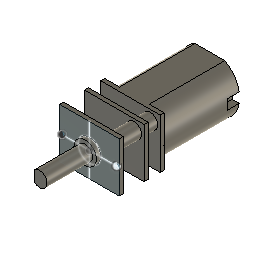
N20 motor (Autodesk Fusion 360 design; units mm, degrees)
Autodesk Fusion 360 part; units mm, degrees
note: some values were not read from the file. Set by a fixed rule: which sketch regions a step uses.
sketch "Sketch1" plane through (0, 0, 0) normal (0, 1, 0) x (1, 0, 0)
  line L0 (0, 0) -> (12, 0)
  line L1 (0, 0) -> (0, -10)
  line L2 (12, 0) -> (12, -10)
  line L3 (12, -10) -> (0, -10)
  line L4 (12, -10) -> (9, -10)
  arc A0 (9, -10) -> (9, 0) centre (6.3333, -5) ccw
  line L5 (0, -10) -> (3, -10)
  arc A1 (3, 0) -> (3, -10) centre (5.6667, -5) ccw
  dimension "d3" = 12
  dimension "d4" = 10
  dimension "d5" = 3
  dimension "d6" = 3
  constraint coincident L0.start L1.start
  constraint horizontal L0
  constraint perpendicular L0 L1
  constraint perpendicular L0 L2
  constraint perpendicular L1 L3
  constraint perpendicular L2 L4
  constraint tangent L2 A0
  constraint coincident L0 A0.end
  constraint perpendicular L1 L5
  constraint tangent L1 A1
  constraint coincident L0 A1.start
  measures "d3" distance of L0.start L0.end
  measures "d4" distance of L0.start L1.end
  measures "d5" distance of L2.end L4.end
  measures "d6" distance of L1.end L5.end
extrude "Extrude1" add sketch "Sketch1" along normal blind 15.2 contours L0 L3 A0 A1 makes body 1
sketch "Sketch2" plane through (0, 0, 0) normal (0, -1, 0) x (1, 0, 0)
  arc A0 (9, 0) -> (9, 10) centre (6.3333, 5) ccw
  line L0 (9, 10) -> (3, 10)
  arc A1 (3, 10) -> (3, 0) centre (5.6667, 5) ccw
  line L1 (3, 0) -> (9, 0)
  line L2 (0, 10) -> (12, 10)
  line L3 (12, 10) -> (12, 0)
  line L4 (12, 0) -> (0, 0)
  line L5 (0, 0) -> (0, 10)
  constraint parallel L0 L2
  constraint perpendicular L2 L3
  constraint coincident L4.end L5.start
  constraint perpendicular L3 L4
  constraint perpendicular L2 L5
extrude "Extrude2" add sketch "Sketch2" along normal blind 0.8 bodies 1
sketch "Sketch3" plane through (0, -0.8, 0) normal (0, -1, 0) x (1, 0, 0)
  line L0 (0, 0) -> (12, 0)
  line L1 (12, 0) -> (12, 10)
  line L2 (12, 10) -> (0, 10)
  line L3 (0, 10) -> (0, 0)
  circle A0 centre (2, 2) radius 1.5
  circle A1 centre (10, 8) radius 1.5
  dimension "d11" = 3
  dimension "d12" = 3
  measures "d11" diameter of A0
  measures "d12" diameter of A1
extrude "Extrude3" add sketch "Sketch3" along normal blind 2.45 contours A0 | A1 bodies 1
sketch "Sketch4" plane through (0, -3.25, 0) normal (0, -1, 0) x (1, 0, 0)
  circle A0 centre (2, 2) radius 1.5
  line L0 (0, 10) -> (12, 10)
  line L1 (12, 10) -> (12, 0)
  line L2 (12, 0) -> (0, 0)
  line L3 (0, 0) -> (0, 10)
  constraint horizontal L0
  constraint vertical L1
  constraint horizontal L2
  constraint vertical L3
extrude "Extrude4" add sketch "Sketch4" along normal blind 0.8 separate body makes body 2
extrude "Extrude5" add 1 faces at (1.5, -3.25, 2.6802) along direction (0, -1, 0) blind 0.8 on bodies 1 bodies 1 2
sketch "Sketch5" plane through (0, -4.05, 0) normal (0, -1, 0) x (1, 0, 0)
  line L0 (0, 0) -> (12, 0)
  line L1 (12, 0) -> (12, 10)
  line L2 (12, 10) -> (0, 10)
  line L3 (0, 10) -> (0, 0)
  circle A0 centre (2, 2) radius 1.5
  circle A1 centre (10, 8) radius 1.5
  dimension "d19" = 3
  dimension "d20" = 3
  measures "d19" diameter of A0
  measures "d20" diameter of A1
extrude "Extrude6" add sketch "Sketch5" along normal blind 4.2 contours A0 | A1 bodies 1
sketch "Sketch6" plane through (0, -8.25, 0) normal (0, -1, 0) x (1, 0, 0)
  circle A0 centre (10, 8) radius 1.5
  line L0 (0, 10) -> (12, 10)
  line L1 (12, 10) -> (12, 0)
  line L2 (12, 0) -> (0, 0)
  line L3 (0, 0) -> (0, 10)
  constraint horizontal L0
  constraint vertical L1
  constraint horizontal L2
  constraint vertical L3
extrude "Extrude7" add sketch "Sketch6" along normal blind 0.8 contours A0 | L0 L1 L2 L3 bodies 1
sketch "Sketch7" plane through (0, -9.05, 0) normal (0, -1, 0) x (1, 0, 0)
  line L0 (0, 0) -> (12, 0)
  line L1 (12, 0) -> (12, 10)
  line L2 (12, 10) -> (0, 10)
  line L3 (0, 10) -> (0, 0)
  line L4 (0, 5) -> (12, 5)
  line L5 (6, 10) -> (6, 0)
  circle A0 centre (6, 5) radius 2.25
  circle A1 centre (0.5, 5) radius 0.35
  circle A2 centre (11.5, 5) radius 0.35
  dimension "d25" = 4.5
  dimension "d26" = 0.7
  constraint midpoint L3 L4.start
  constraint midpoint L1 L4.end
  constraint midpoint L2 L5.start
  constraint midpoint L0 L5.end
  constraint midpoint L4 A0.centre
  constraint coincident L4 A1.centre
  constraint symmetric L5 A1 A2
  measures "d25" diameter of A0
  measures "d26" diameter of A1
extrude "Extrude8" cut sketch "Sketch7" against normal blind 2 contours L4 A1 | L4 A1 | L4 A2 | L4 A2 bodies 1
extrude "Extrude9" add sketch "Sketch7" along normal blind 0.87 contours L4 L5 A0 | L4 L5 A0 | L4 L5 A0 | L4 L5 A0 bodies 1
sketch "Sketch8" plane through (0, -9.92, 0) normal (0, -1, 0) x (1, 0, 0)
  circle A0 centre (6, 5) radius 2.25
  line L0 (7.5, 5) -> (5, 5)
  line L1 (5, 5) -> (5, 6.118)
  line L2 (5, 5) -> (5, 3.882)
  arc A1 (5, 3.882) -> (5, 6.118) centre (6, 5) ccw
  dimension "d31" = 3
  dimension "d32" = 2.5
  constraint concentric A0 A1
  constraint coincident L0.start A1
  constraint horizontal L0
  constraint perpendicular L0 L1
  constraint perpendicular L0 L2
  measures "d31" diameter of A1
  measures "d32" distance of L0.start L0.end
extrude "Extrude10" add sketch "Sketch8" along normal blind 9.17 contours L0 L2 A1 | L0 L1 A1 bodies 1
sketch "Sketch9" plane through (0, 15.2, 0) normal (0, 1, 0) x (-1, 0, 0)
  arc A0 (-9, 10) -> (-9, 0) centre (-6.3333, 5) ccw
  line L0 (-9, 0) -> (-3, 0)
  arc A1 (-3, 0) -> (-3, 10) centre (-5.6667, 5) ccw
  line L1 (-3, 10) -> (-9, 10)
  circle A2 centre (-6, 5) radius 2.5
  line L2 (0, 5) -> (-1.5, 5)
  line L3 (-1.5, 5) -> (-1.5, 4)
  line L4 (0, 5) -> (0, 6)
  line L5 (0, 6) -> (-1.5, 6)
  line L6 (-1.5, 6) -> (-1.5, 4)
  line L7 (-1.5, 4) -> (0, 4)
  line L8 (0, 4) -> (0, 6)
  line L9 (-6, 10) -> (-6, 0)
  line L10 (-10.5, 6) -> (-10.5, 4)
  line L11 (-12, 4) -> (-12, 6)
  line L12 (-10.5, 4) -> (-12, 4)
  line L13 (-12, 6) -> (-10.5, 6)
  dimension "d35" = 5
  dimension "d36" = 1.5
  dimension "d37" = 1
  dimension "d38" = 1
  constraint midpoint A1 L2.start
  constraint horizontal L2
  constraint perpendicular L2 L3
  constraint perpendicular L2 L4
  constraint horizontal L5
  constraint vertical L6
  constraint horizontal L7
  constraint vertical L8
  constraint symmetric L3.end L9 L10.end
  constraint symmetric L4.end L9 L11.end
  constraint symmetric L5.end L9 L10.start
  constraint symmetric L7.end L9 L11.start
  measures "d35" diameter of A2
  measures "d36" distance of L2.start L2.end
  measures "d37" distance of L2.end L3.end
  measures "d38" distance of L2.start L4.end
extrude "Extrude11" add sketch "Sketch9" along normal blind 0.9 contours A2 L9 | A2 L9 bodies 1
extrude "Extrude12" cut sketch "Sketch9" against normal blind 2.37 contours A0 L10 L12 L13 | A1 L2 L5 L6 | A1 L2 L3 L6 L7 bodies 1
sketch "Sketch10" plane through (0, 15.2, 0) normal (0, 1, 0) x (-1, 0, 0)
  line L0 (-0.0889, 4) -> (-1.5, 4)
  line L1 (-1.5, 4) -> (-1.5, 6)
  line L2 (-1.5, 6) -> (-0.0889, 6)
  arc A0 (-0.0889, 6) -> (-3, 10) centre (-5.6667, 5) ccw
  line L3 (-3, 10) -> (-9, 10)
  arc A1 (-9, 10) -> (-11.9111, 6) centre (-6.3333, 5) ccw
  line L4 (-11.9111, 6) -> (-10.5, 6)
  line L5 (-10.5, 6) -> (-10.5, 4)
  line L6 (-10.5, 4) -> (-11.9111, 4)
  arc A2 (-11.9111, 4) -> (-9, 0) centre (-6.3333, 5) ccw
  line L7 (-9, 0) -> (-3, 0)
  arc A3 (-3, 0) -> (-0.0889, 4) centre (-5.6667, 5) ccw
  circle A4 centre (-6, 5) radius 2.5
  line L8 (-3.5, 5) -> (-2.39, 5)
  line L9 (-2.39, 5) -> (-2.39, 4.25)
  line L10 (-2.39, 4.25) -> (-2.09, 4.25)
  line L11 (-2.09, 4.25) -> (-2.09, 5)
  line L12 (0, 5) -> (-12, 5)
  line L13 (-3.5, 5) -> (-2.39, 5)
  line L14 (-2.39, 5.75) -> (-2.09, 5.75)
  line L15 (-2.09, 5.75) -> (-2.09, 5)
  line L16 (-2.39, 5) -> (-2.39, 5.75)
  line L17 (-6, 10) -> (-6, 0)
  line L18 (-9.61, 5) -> (-9.61, 4.25)
  line L19 (-9.91, 4.25) -> (-9.91, 5)
  line L20 (-9.61, 4.25) -> (-9.91, 4.25)
  line L21 (-12, 5) -> (0, 5)
  line L22 (-9.61, 5.75) -> (-9.91, 5.75)
  line L23 (-9.61, 5) -> (-9.61, 5.75)
  line L24 (-9.91, 5.75) -> (-9.91, 5)
  dimension "d43" = 1.11
  dimension "d44" = 0.75
  dimension "d45" = 0.3
  constraint coincident A4 L8.start
  constraint perpendicular L1 L8
  constraint perpendicular L8 L9
  constraint perpendicular L9 L10
  constraint perpendicular L10 L11
  constraint symmetric L8.start L12 L13.start
  constraint symmetric L8.end L12 L9.start
  constraint symmetric L9.end L12 L14.start
  constraint symmetric L10.end L12 L14.end
  constraint symmetric L11.end L12 L15.end
  constraint symmetric L8.end L17 L18.start
  constraint symmetric L9.end L17 L18.end
  constraint symmetric L10.end L17 L19.start
  constraint symmetric L11.end L17 L19.end
  constraint symmetric L12.start L17 L12.end
  constraint symmetric L12.end L17 L12.start
  constraint symmetric L14.start L17 L22.start
  constraint symmetric L14.end L17 L22.end
  measures "d43" distance of L8.start L8.end
  measures "d44" distance of L8.end L9.end
  measures "d45" distance of L9.end L10.end
extrude "Extrude13" add sketch "Sketch10" along normal blind 1.31 contours L9 L10 L11 L12 L21 | L12 L14 L15 L16 L21 | L12 L18 L19 L20 L21 | L12 L21 L22 L23 L24 bodies 1
sketch "Sketch11" plane through (2.09, 0, 0) normal (-1, 0, 0) x (0, -1, 0)
  line L0 (-15.2, 4.25) -> (-15.2, 5.75)
  line L1 (-15.2, 5.75) -> (-16.51, 5.75)
  line L2 (-16.51, 5.75) -> (-16.51, 4.25)
  line L3 (-16.51, 4.25) -> (-15.2, 4.25)
  circle A0 centre (-15.8, 5) radius 0.4
extrude "Extrude14" cut sketch "Sketch11" against normal blind 0.7 contours A0 bodies 1
sketch "Sketch12" plane through (9.91, 0, 0) normal (1, 0, 0) x (0, 1, 0)
  line L0 (15.2, 5.75) -> (15.2, 4.25)
  line L1 (15.2, 4.25) -> (16.51, 4.25)
  line L2 (16.51, 4.25) -> (16.51, 5.75)
  line L3 (16.51, 5.75) -> (15.2, 5.75)
  circle A0 centre (15.8, 5) radius 0.4
extrude "Extrude15" cut sketch "Sketch12" against normal blind 0.4 contours A0 bodies 1
fillet "Fillet1" radius 0.4 2 edges at (9.76, 16.51, 4.25) (9.76, 16.51, 5.75) on bodies 1
fillet "Fillet2" radius 0.4 2 edges at (2.24, 16.51, 4.25) (2.24, 16.51, 5.75) on bodies 1
sketch "Sketch13" plane through (0, 16.1, 0) normal (0, 1, 0) x (-1, 0, 0)
  circle A0 centre (-6, 5) radius 2.5
  circle A1 centre (-6, 5) radius 0.93
  dimension "d56" = 1.86
  constraint concentric A0 A1
  measures "d56" diameter of A1
extrude "Extrude16" cut sketch "Sketch13" against normal blind 0.5 contours A1 bodies 1
equation "d5 = ( 12 / 4 ) * 1 mm"
equation "d7 = 16 mm - 0.8 mm"
equation "d44 = ( 1.5 / 2 ) * 1 mm"
